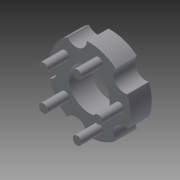
# Autodesk Inventor part: Ротор цевков
Saved by Autodesk Inventor 2013 (Build 170138000, 138)
## iProperties
Created: 2014-04-30
Part Number: Ротор цевков
Material: Типовые
Document SubType Name: Modeling
Designer: HP1
Density: 1 g/cm^3
Mass: 7.76673 g
Surface Area: 39.9048 cm^2
Volume: 7.76673 cm^3
Author: HP1
Autodesk Inventor part; units mm, degrees
ref_plane "YZ Plane" through (0, 0, 0) normal (1, 0, 0) x (0, 1, 0)
ref_plane "XZ Plane" through (0, 0, 0) normal (0, 1, 0) x (-1, 0, 0)
ref_plane "XY Plane" through (0, 0, 0) normal (0, 0, 1) x (1, 0, 0)
sketch "Эскиз1" plane through (0, 0, 0) normal (0, 1, 0) x (-1, 0, 0)
  circle A0 centre (0, 0) radius 9.5
  circle A1 centre (0, 0) radius 30
  circle A2 centre (0, 0) radius 20 construction
  circle A3 centre (19.9999, 0) radius 5
  circle A4 centre (6.1803, 19.021) radius 5
  circle A5 centre (-16.1803, 11.7557) radius 5
  circle A6 centre (-16.1803, -11.7557) radius 5
  circle A7 centre (6.1803, -19.021) radius 5
  dimension "d0" = 19
  dimension "d1" = 60
  dimension "d2" = 40
  dimension "d3" = 10
  dimension "d6" = 360
  constraints: 8 centre point, 11 other
  measures "d0" diameter of A0
  measures "d1" diameter of A1
  measures "d2" diameter of A2
  measures "d3" diameter of A3
extrude "Выдавливание1" add sketch "Эскиз1" along normal blind 10
sketch "Эскиз2" plane through (0, 10, 0) normal (0, 1, 0) x (1, 0, 0)
  circle A0 centre (-6.1803, 19.021) radius 5 projected
  circle A1 centre (16.1803, 11.7557) radius 5 projected
  circle A2 centre (16.1803, -11.7557) radius 5 projected
  circle A3 centre (-6.1803, -19.021) radius 5 projected
  circle A4 centre (-19.9999, 0) radius 5 projected
  circle A5 centre (0, 0) radius 30 projected
  circle A6 centre (0, 0) radius 19
  dimension "d15" = 38
  constraints: 1 centre point
  measures "d15" diameter of A6
extrude "Выдавливание2" cut sketch "Эскиз2" against normal blind 10
sketch "Эскиз3" plane through (0, 10, 0) normal (0, 1, 0) x (1, 0, 0)
  circle A0 centre (0, 0) radius 9.5 projected
  circle A1 centre (14, 0) radius 2
  circle A2 centre (4.3262, 13.3148) radius 2
  circle A3 centre (-11.3262, 8.229) radius 2
  circle A4 centre (-11.3262, -8.229) radius 2
  circle A5 centre (4.3262, -13.3148) radius 2
  dimension "d17" = 4
  dimension "d18" = 14
  dimension "d21" = 360
  constraints: 5 centre point, 11 other
  measures "d17" diameter of A1
  measures "d18" distance of A0.centre A1.centre
extrude "Выдавливание3" add sketch "Эскиз3" against normal blind 20 contours A1 | A2 | A3 | A4 | A5
